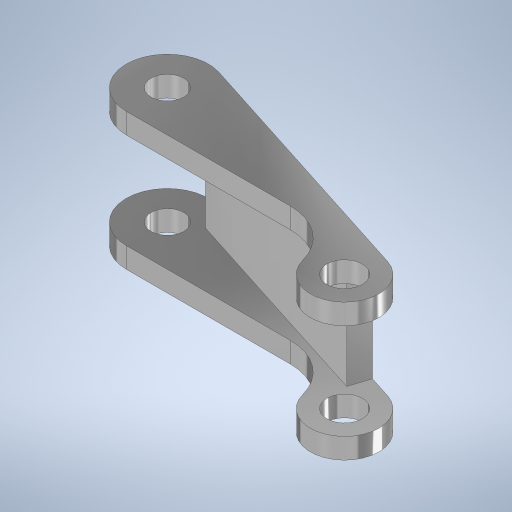
# Autodesk Inventor part: Lever for inset hinge
Saved by Autodesk Inventor 2024 (Build 280153000, 153)
## iProperties
Created: 2008-03-26
Part Number: Lever for inset hinge
Document SubType Name: Modeling
Designer: G.K.
Material: Steel
Description: Lever for inset hinge
Authority: Design by UAB Čeli APS
Mass: 3.34964 g
Surface Area: 7.60263 cm^2
Volume: 0.426705 cm^3
Density: 7.85 g/cm^3
Appearance: Chrome - Polished
Mase: 0.00334964
Autodesk Inventor part; units mm, degrees
ref_plane "YZ Plane" through (0, 0, 0) normal (1, 0, 0) x (0, 1, 0)
ref_plane "XZ Plane" through (0, 0, 0) normal (0, 1, 0) x (-1, 0, 0)
sketch "Sketch1" plane through (0, 0, 0) normal (0, 0, 1) x (1, 0, 0)
  circle A0 centre (17.6, 46.7) radius 1.2
  circle A1 centre (35.8812, 41.3663) radius 1.3
  arc A2 (18.5156, 49.5569) -> (17.5984, 43.7) centre (17.6, 46.7) ccw
  arc A3 (33.4647, 40.7254) -> (36.6442, 43.747) centre (35.8812, 41.3663) ccw
  line L0 (18.5156, 49.5569) -> (36.6442, 43.747)
  line L1 (17.5984, 43.7) -> (29.5984, 43.7)
  arc A4 (33.4647, 40.7254) -> (29.5984, 43.7) centre (29.5984, 39.7) ccw
  point P0 (0, 0)
  dimension "d0" = 5
  dimension "d1" = 3
  dimension "d3" = 4
  dimension "d14" = 12
  constraints: 6 point on circle, 5 centre point, 5 end point, 4 tangent, 2 coincident, 1 horizontal, 4 other
  measures "d0" diameter of A3
  measures "d1" radius of A2
  measures "d3" radius of A4
  measures "d14" distance of L1.start L1.end
extrude "Extrusion1" add sketch "Sketch1" along normal mid plane 10
ref_plane "Work Plane1" through (36.1864, 42.3186, 5) normal (0.3051918, 0.9522909, 0) x (0.9522909, -0.3051918, 0)
sketch "Sketch2" plane through (36.1864, 42.3186, 5) normal (0.3051918, 0.9522909, 0) x (0.9522909, -0.3051918, 0)
  line L0 (8.5468, 5) -> (-28.0353, 5) projected
  line L1 (-22.0368, 8.5) -> (2.5, 8.5)
  line L2 (2.5, 8.5) -> (2.5, 1.5)
  line L3 (2.5, 1.5) -> (-22.0368, 1.5)
  line L4 (-22.0368, 1.5) -> (-22.0368, 8.5)
  line L5 (2.5, 10) -> (2.5, 0) projected
  line L6 (-22.0368, 10) -> (-22.0368, 0) projected
  point P0 (-21.5447, 5)
  dimension "d7" = 7
  constraints: 8 end point, 2 collinear, 2 parallel, 1 horizontal, 1 perpendicular, 1 other
  measures "d7" distance of L3.end L1.start
extrude "Extrusion2" cut sketch "Sketch2" against normal through all
sketch "Sketch3" plane through (36.1864, 42.3186, 5) normal (-0.3051918, -0.9522909, 0) x (0.9522909, -0.3051918, 0)
  line L0 (-21.6349, -8.5) -> (-21.6349, -1.5) projected
  line L1 (-21.6349, -8.5) -> (2.2913, -8.5) projected
  line L2 (2.2913, -1.5) -> (2.2913, -8.5) projected
  line L3 (-21.6349, -1.5) -> (-17.6349, -1.5)
  line L4 (-17.6349, -1.5) -> (-17.6349, -8.5)
  line L5 (-17.6349, -8.5) -> (-21.6349, -8.5)
  line L6 (-21.6349, -8.5) -> (-21.6349, -1.5)
  line L7 (2.2913, -1.5) -> (-1.7087, -1.5)
  line L8 (-1.7087, -1.5) -> (-1.7087, -8.5)
  line L9 (-1.7087, -8.5) -> (2.2913, -8.5)
  line L10 (2.2913, -8.5) -> (2.2913, -1.5)
  point P0 (-21.5447, -5)
  dimension "d10" = 4
  dimension "d11" = 4
  constraints: 16 end point, 4 parallel, 2 horizontal, 2 perpendicular, 2 point on line
  measures "d10" distance between parallel lines of L4 L6
  measures "d11" distance between parallel lines of L2 L8
extrude "Extrusion3" cut sketch "Sketch3" against normal through all
body "Solid1"
